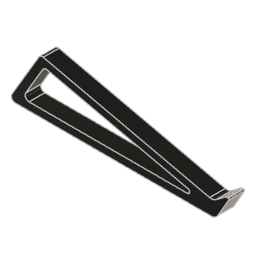
Laptop stand concept (Autodesk Fusion 360 design; units mm, degrees)
Autodesk Fusion 360 part; units mm, degrees
sketch "Sketch1" plane through (0, 0, 0) normal (0, 1, 0) x (1, 0, 0)
  line L0 (4.4636, -7.5457) -> (38.8694, -65.7079)
  line L1 (44.2942, -68.0348) -> (255.4212, -19.4495)
  line L2 (263.7339, -21.2478) -> (274.5501, -29.5094)
  line L3 (278.9981, -30.5359) -> (277.5851, -30.5359)
  arc A0 (8.7671, 0) -> (4.4636, -7.5457) centre (8.7671, -5) ccw
  arc A1 (38.8694, -65.7079) -> (44.2942, -68.0348) centre (43.1729, -63.1622) ccw
  arc A2 (263.7339, -21.2478) -> (255.4212, -19.4495) centre (257.6638, -29.1948) ccw
  arc A3 (274.5501, -29.5094) -> (277.5851, -30.5359) centre (277.5851, -25.5359) ccw
  arc A4 (278.9981, -30.5359) -> (279.8234, -28.9712) centre (278.9981, -29.5359) ccw
  line L4 (8.7671, 0) -> (257.3233, 0)
  line L5 (279.8234, -28.9712) -> (265.9836, -5)
  line L6 (279.8234, -28.9712) -> (314.5624, -28.9712) construction
  arc A5 (265.9836, -5) -> (257.3233, 0) centre (257.3233, -10) ccw
  line L7 (26.3012, -10) -> (227.973, -10)
  line L8 (21.9978, -17.5457) -> (43.7532, -54.3227)
  line L9 (49.1779, -56.6496) -> (228.4216, -15.4014)
  arc A6 (43.7532, -54.3227) -> (49.1779, -56.6496) centre (48.0566, -51.777) ccw
  arc A7 (26.3012, -10) -> (21.9978, -17.5457) centre (26.3012, -15) ccw
  line L10 (229.973, -13.4524) -> (229.973, -12)
  arc A8 (228.4216, -15.4014) -> (229.973, -13.4524) centre (227.973, -13.4524) ccw
  arc A9 (229.973, -12) -> (227.973, -10) centre (227.973, -12) ccw
  point P0 (40.731, -68.8548)
  point P1 (260, -18.3958)
  point P2 (275.894, -30.5359)
  point P3 (280.894, -30.5359)
  point P4 (308.7671, 0)
  dimension "d7" = 80
  dimension "d8" = 225
  dimension "d9" = 20
  dimension "d11" = 5
  dimension "d12" = 107.647
  dimension "d13" = 5
  dimension "d14" = 5
  dimension "d15" = 10
  dimension "d16" = 5
  dimension "d17" = 1
  dimension "d25" = 300
  dimension "d26" = 120
  dimension "d27" = 10
  dimension "d29" = 5
  dimension "d30" = 5
  dimension "d31" = 2
  constraint coincident origin L0
  constraint tangent L0 A0
  constraint coincident P0 L0
  constraint coincident P0 L1
  constraint tangent L0 A1
  constraint tangent L1 A1
  constraint coincident P1 L1
  constraint coincident P1 L2
  constraint tangent L1 A2
  constraint tangent L2 A2
  constraint coincident P2 L3
  constraint coincident P2 L2
  constraint tangent L3 A3
  constraint tangent L2 A3
  constraint coincident P3 L3
  constraint tangent L3 A4
  constraint coincident A0.start L4.start
  constraint horizontal L4
  constraint horizontal L6
  constraint coincident A4.end L5.start
  constraint coincident P4 L4
  constraint tangent L5 A5
  constraint tangent L4 A5
  constraint tangent L9 A6
  constraint tangent L8 A6
  constraint tangent L8 A7
  constraint tangent L7 A7
  constraint perpendicular L7 L10
  constraint tangent L9 A8
  constraint tangent L10 A8
  constraint tangent L7 A9
  constraint tangent L10 A9
  constraint equal A8 A9
  measures "d7" distance of origin P0
  measures "d8" distance of P0 P1
  measures "d9" distance of P1 P2
  measures "d11" distance of P2 P3
  measures "d12" angle of L0 L1
  measures "d13" radius of A0
  measures "d14" radius of A1
  measures "d15" radius of A2
  measures "d16" radius of A3
  measures "d17" radius of A4
  measures "d25" distance of A0.start P4
  measures "d26" angle of L5 L6
  measures "d27" radius of A5
  measures "d29" radius of A6
  measures "d30" radius of A7
  measures "d31" radius of A8
extrude "Extrude1" add sketch "Sketch1" along normal blind 20 contours L0 L1 L2 L3 A0 A1 A2 A3 A4 L4 L5 A5 | L7 L8 L9 A6 A7 L10 A8 A9 makes body 1
copy_body "CopyPasteBodies1" bodies 1 makes body 2
move_body "Move1" bodies 2 to x (1, 0, 0) y (0, 1, 0) z (0, 0, 1) at (0, 110, 0)
extrude "Extrude2" cut sketch "Sketch1" along normal blind 200 contours L7 L8 L9 A6 A7 L10 A8 A9 bodies 1 2
delete_body "RemoveBody1" bodies 2
